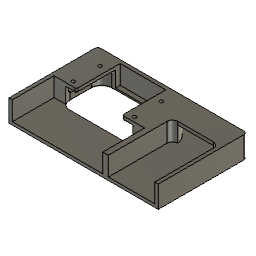
co2_o2_fascia (Autodesk Fusion 360 design; units mm, degrees)
part number: 2026-03-11-11-56-11-354
Autodesk Fusion 360 part; units mm, degrees
note: some values were not read from the file. Set by a fixed rule: which sketch regions a step uses.
sketch "Sketch1" plane through (0, 0, 0) normal (0, 0, 1) x (1, 0, 0)
  line L0 (0, 0) -> (95, 0)
  line L1 (95, 0) -> (95, 56.5)
  line L2 (95, 56.5) -> (0, 56.5)
  line L3 (0, 56.5) -> (0, 0)
  dimension "d1" = 95
  dimension "d2" = 56.5
  constraint horizontal L0
  constraint vertical L1
  constraint horizontal L2
  constraint vertical L3
  constraint coincident L0.start L3.end
  measures "d1" distance of L0.start L0.end
  measures "d2" distance of L0.start L2.end
extrude "Extrude1" add sketch "Sketch1" along normal blind 14
sketch "Sketch2" plane through (0, 0, 14) normal (0, 0, 1) x (-1, 0, 0)
  line L0 (0, -56.5) -> (0, 0)
  line L1 (0, 0) -> (-95, 0)
  line L2 (-95, 0) -> (-95, -56.5)
  line L3 (-95, -56.5) -> (0, -56.5)
  line L4 (-2.25, -26.5) -> (-92.75, -26.5)
  line L5 (-92.75, -26.5) -> (-92.75, 0.5)
  line L6 (-92.75, 0.5) -> (-2.25, 0.5)
  line L7 (-2.25, 0.5) -> (-2.25, -26.5)
  line L8 (-92.75, -26.5) -> (-60, -26.5)
  dimension "d5" = 90.5
  dimension "d6" = 27
  dimension "d7" = 30
  dimension "d8" = 2.25
  constraint horizontal L4
  constraint vertical L5
  constraint horizontal L6
  constraint vertical L7
  constraint horizontal L8
  measures "d5" distance of L4.start L4.end
  measures "d6" distance of L4.start L6.end
  measures "d7" distance of L3 L4
  measures "d8" distance of L0 L7
extrude "Extrude2" cut sketch "Sketch2" against normal blind 12 contours L1 L4 L5 L7 L8 | L1 L5 L6 L7
sketch "Sketch3" plane through (0, 0, 14) normal (0, 0, 1) x (-1, 0, 0)
  line L0 (-92.75, -26.5) -> (-92.75, 0)
  line L1 (-92.75, 0) -> (-95, 0)
  line L2 (-95, 0) -> (-95, -56.5)
  line L3 (-95, -56.5) -> (0, -56.5)
  line L4 (0, -56.5) -> (0, 0)
  line L5 (0, 0) -> (-2.25, 0)
  line L6 (-2.25, 0) -> (-2.25, -26.5)
  line L7 (-2.25, -26.5) -> (-92.75, -26.5)
  point P0 (-11.5, -46.5)
  point P1 (-50.5, -46.5)
  point P2 (-11.5, -29.5)
  point P3 (-50.5, -29.5)
  dimension "d11" = 10
  dimension "d12" = 11.5
  dimension "d15" = -39
  dimension "d16" = 17
  measures "d11" distance of L3 P0
  measures "d12" distance of L4 P0
hole "Hole1" at (50.5, 46.5, 14) at (50.5, 29.5, 14) at (11.5, 29.5, 14) at (11.5, 46.5, 14) direction (0, 0, -1) diameter 2.2 end through all
sketch "Sketch4" plane through (0, 0, 0) normal (0, 0, -1) x (1, 0, 0)
  circle A0 centre (11.5, -29.5) radius 1.1
  circle A1 centre (50.5, -46.5) radius 1.1
  circle A2 centre (50.5, -29.5) radius 1.1
  circle A3 centre (11.5, -46.5) radius 1.1
  line L0 (0, 0) -> (0, -56.5)
  line L1 (0, -56.5) -> (95, -56.5)
  line L2 (95, -56.5) -> (95, 0)
  line L3 (95, 0) -> (0, 0)
  line L4 (47.75, -51.275) -> (14.2, -51.275)
  line L5 (7.7, -44.775) -> (7.7, -31.225)
  line L6 (14.2, -24.725) -> (47.75, -24.725)
  line L7 (54.25, -31.225) -> (54.25, -44.775)
  arc A4 (47.75, -51.275) -> (54.25, -44.775) centre (47.75, -44.775) ccw
  arc A5 (7.7, -44.775) -> (14.2, -51.275) centre (14.2, -44.775) ccw
  arc A6 (14.2, -24.725) -> (7.7, -31.225) centre (14.2, -31.225) ccw
  arc A7 (54.25, -31.225) -> (47.75, -24.725) centre (47.75, -31.225) ccw
  point P0 (54.25, -51.275)
  point P1 (7.7, -51.275)
  point P2 (54.25, -24.725)
  dimension "d19" = 46.55
  dimension "d20" = 26.55
  dimension "d21" = 40.75
  dimension "d22" = 4.775
  dimension "d35" = 6.5
  constraint horizontal L4
  constraint vertical L5
  constraint horizontal L6
  constraint vertical L7
  constraint coincident P0 L7
  constraint coincident P0 L4
  constraint tangent L7 A4
  constraint tangent L4 A4
  constraint coincident P1 L4
  constraint coincident P1 L5
  constraint tangent L4 A5
  constraint tangent L5 A5
  constraint equal A4 A5
  constraint tangent L5 A6
  constraint tangent L6 A6
  constraint equal A4 A6
  constraint coincident P2 L6
  constraint coincident P2 L7
  constraint tangent L6 A7
  constraint tangent L7 A7
  constraint equal A4 A7
  measures "d19" distance of P0 P1
  measures "d20" distance of P0 P2
  measures "d21" distance of L2 L7
  measures "d22" distance of A1.centre L4
  measures "d35" radius of A4
extrude "Extrude3" cut sketch "Sketch4" against normal blind 11 contours L4 L5 L6 L7 A4 A5 A6 A7
sketch "Sketch5" plane through (0, 0, 0) normal (-1, 0, 0) x (0, -1, 0)
  line L0 (-56.5, 0) -> (0, 0)
  line L1 (0, 0) -> (0, 14)
  line L2 (0, 14) -> (-56.5, 14)
  line L3 (-56.5, 14) -> (-56.5, 0)
sketch "Sketch7" plane through (0, 0, 0) normal (-1, 0, 0) x (0, -1, 0)
  line L0 (-32, 13) -> (-44, 13)
  line L1 (-46, 11) -> (-46, 7)
  line L2 (-44, 5) -> (-32, 5)
  line L3 (-30, 7) -> (-30, 11)
  line L4 (-56.5, 14) -> (-56.5, 0)
  arc A0 (-32, 5) -> (-30, 7) centre (-32, 7) ccw
  arc A1 (-46, 7) -> (-44, 5) centre (-44, 7) ccw
  line L5 (-56.5, 0) -> (0, 0)
  arc A2 (-30, 11) -> (-32, 13) centre (-32, 11) ccw
  arc A3 (-44, 13) -> (-46, 11) centre (-44, 11) ccw
  point P0 (-30, 13)
  point P1 (-46, 13)
  point P2 (-30, 5)
  dimension "d30" = 16
  dimension "d31" = 8
  dimension "d32" = 10.5
  dimension "d42" = 2
  dimension "d140" = 5
  dimension "d141" = 2
  dimension "d142" = 2
  constraint horizontal L0
  constraint vertical L1
  constraint horizontal L2
  constraint vertical L3
  constraint coincident P2 L3
  constraint coincident P2 L2
  constraint tangent L3 A0
  constraint tangent L2 A0
  constraint tangent L2 A1
  constraint tangent L1 A1
  constraint equal A0 A1
  constraint coincident P0 L3
  constraint coincident P0 L0
  constraint tangent L3 A2
  constraint tangent L0 A2
  constraint coincident P1 L0
  constraint coincident P1 L1
  constraint tangent L0 A3
  constraint tangent L1 A3
  measures "d30" distance of P0 P1
  measures "d31" distance of P0 P2
  measures "d32" distance of L1 L4
  measures "d42" radius of A0
  measures "d140" distance of L2 L5
  measures "d141" radius of A2
  measures "d142" radius of A3
extrude "Extrude5" cut sketch "Sketch7" against normal blind 8.5
sketch "Sketch8" plane through (0, 0, 14) normal (0, 0, 1) x (-1, 0, 0)
  line L0 (0, 0) -> (-2.25, 0)
  line L1 (-2.25, 0) -> (-2.25, -26.5)
  line L2 (-2.25, -26.5) -> (-92.75, -26.5)
  line L3 (-92.75, -26.5) -> (-92.75, 0)
  line L4 (-92.75, 0) -> (-95, 0)
  line L5 (-95, 0) -> (-95, -56.5)
  line L6 (-95, -56.5) -> (0, -56.5)
  line L7 (0, -56.5) -> (0, 0)
  circle A0 centre (-11.5, -29.5) radius 1.1
  circle A1 centre (-50.5, -46.5) radius 1.1
  circle A2 centre (-50.5, -29.5) radius 1.1
  circle A3 centre (-11.5, -46.5) radius 1.1
  line L8 (-16.5, -54.25) -> (-45.5, -54.25)
  line L9 (-45.5, -54.25) -> (-45.5, -14.25)
  line L10 (-45.5, -14.25) -> (-16.5, -14.25)
  line L11 (-16.5, -14.25) -> (-16.5, -54.25)
  dimension "d36" = 29
  dimension "d37" = 40
  dimension "d38" = 2.25
  dimension "d39" = 49.5
  constraint horizontal L8
  constraint vertical L9
  constraint horizontal L10
  constraint vertical L11
  measures "d36" distance of L8.start L8.end
  measures "d37" distance of L8.start L10.end
  measures "d38" distance of L6 L8
  measures "d39" distance of L5 L9
extrude "Extrude6" cut sketch "Sketch8" against normal blind 2.5 contours L2 L8 L9 L11 | L2 L9 L10 L11
fillet "Fillet1" radius 2 1 edges at (95, 56.5, 7)
fillet "Fillet2" radius 2 1 edges at (0, 56.5, 7)
fillet "Fillet3" radius 1 8 edges at (7.7, 38, 0) (9.6038, 26.6288, 0) (30.975, 24.725, 0) (52.3462, 26.6288, 0) (54.25, 38, 0) (52.3462, 49.3712, 0) (30.975, 51.275, 0) (9.6038, 49.3712, 0)
fillet "Fillet4" radius 1 5 edges at (0, 30, 9) (0, 30.5858, 5.5858) (0, 38, 5) (0, 45.4142, 5.5858) (0, 46, 9)
extrude "Extrude13" cut 1 faces at (35.8333, 45, 11.5) along direction (0, 0, -1) blind 9.5
sketch "Sketch13" plane through (0, 0, 14) normal (0, 0, 1) x (-1, 0, 0)
  arc A0 (-2, -56.5) -> (0, -54.5) centre (-2, -54.5) ccw
  line L0 (0, -54.5) -> (0, -44)
  line L1 (0, 0) -> (-2.25, 0)
  line L2 (-2.25, 0) -> (-2.25, -26.5)
  line L3 (-2.25, -26.5) -> (-16.5, -26.5)
  line L4 (-16.5, -26.5) -> (-16.5, -54.25)
  line L5 (-16.5, -54.25) -> (-45.5, -54.25)
  line L6 (-45.5, -54.25) -> (-45.5, -26.5)
  line L7 (-45.5, -26.5) -> (-92.75, -26.5)
  line L8 (-92.75, -26.5) -> (-92.75, 0)
  line L9 (-92.75, 0) -> (-95, 0)
  line L10 (-95, 0) -> (-95, -54.5)
  arc A1 (-95, -54.5) -> (-93, -56.5) centre (-93, -54.5) ccw
  line L11 (-93, -56.5) -> (-2, -56.5)
  circle A2 centre (-11.5, -29.5) radius 1.1
  circle A3 centre (-50.5, -46.5) radius 1.1
  circle A4 centre (-50.5, -29.5) radius 1.1
  circle A5 centre (-11.5, -46.5) radius 1.1
  line L12 (-92.75, -26.5) -> (-63.25, -26.5)
  line L13 (-63.25, -26.5) -> (-63.25, -37.331)
  line L14 (-66.669, -40.75) -> (-89.331, -40.75)
  line L15 (-92.75, -37.331) -> (-92.75, -26.5)
  arc A6 (-66.669, -40.75) -> (-63.25, -37.331) centre (-66.669, -37.331) ccw
  arc A7 (-92.75, -37.331) -> (-89.331, -40.75) centre (-89.331, -37.331) ccw
  line L16 (0, -44) -> (0, -32)
  line L17 (0, -32) -> (0, 0)
  dimension "d107" = 29.5
  dimension "d108" = 15.75
  dimension "d118" = 3.419
  dimension "d119" = 3.419
  constraint horizontal L12
  constraint vertical L13
  constraint horizontal L14
  constraint vertical L15
  constraint coincident L7.end L8.start
  constraint tangent L13 A6
  constraint tangent L14 A6
  constraint tangent L14 A7
  constraint tangent L15 A7
  measures "d107" distance of L7.end L12.end
  measures "d108" distance of L11 L14
  measures "d118" radius of A6
  measures "d119" radius of A7
extrude "Extrude20" cut sketch "Sketch13" against normal blind 12 contours L7 L12 L13 L14 L15 A6 A7
sketch "Sketch16" plane through (0, 40.75, 0) normal (0, -1, 0) x (1, 0, 0)
  line L0 (89.331, 14) -> (66.669, 14)
  line L1 (66.669, 14) -> (66.669, 2)
  line L2 (66.669, 2) -> (89.331, 2)
  line L3 (89.331, 2) -> (89.331, 14)
  line L4 (89.331, 2) -> (66.669, 2)
  line L5 (66.669, 2) -> (66.669, 12)
  line L6 (66.669, 12) -> (89.331, 12)
  line L7 (89.331, 12) -> (89.331, 2)
  dimension "d120" = 10
  constraint horizontal L4
  constraint vertical L5
  constraint horizontal L6
  constraint vertical L7
  constraint coincident L1 L5.end
  constraint coincident L2.end L3.start
  measures "d120" distance of L2.end L6.end
extrude "Extrude23" cut sketch "Sketch16" against normal blind 13.5 contours L1 L2 L3 L4 L5 L6 L7
sketch "Sketch17" plane through (66.669, 0, 0) normal (1, 0, 0) x (0, 1, 0)
  line L0 (40.75, 12) -> (40.75, 2)
  line L1 (40.75, 2) -> (54.25, 2)
  line L2 (54.25, 2) -> (54.25, 12)
  line L3 (54.25, 12) -> (40.75, 12)
  line L4 (54.25, 2) -> (49.25, 2)
  line L5 (49.25, 2) -> (49.25, 12)
  line L6 (49.25, 12) -> (54.25, 12)
  line L7 (54.25, 12) -> (54.25, 2)
  dimension "d123" = 5
  dimension "d124" = 10
  constraint horizontal L4
  constraint vertical L5
  constraint horizontal L6
  constraint vertical L7
  constraint coincident L1.end L2.start
  measures "d123" distance of L1.end L4.end
  measures "d124" distance of L1.end L2.end
extrude "Extrude24" cut sketch "Sketch17" against normal blind 30 contours L1 L2 L3 L4 L5 L6 L7
fillet "Fillet15" radius 10 1 edges at (66.669, 49.25, 7)
sketch "Sketch18" plane through (0, 26.5, 0) normal (0, -1, 0) x (1, 0, 0)
  line L0 (63.25, 2) -> (63.25, 14)
  line L1 (63.25, 14) -> (45.5, 14)
  line L2 (45.5, 14) -> (45.5, 11)
  line L3 (45.5, 11) -> (52.2137, 11)
  line L4 (52.2137, 11) -> (52.2137, 2)
  line L5 (52.2137, 2) -> (63.25, 2)
  line L6 (59.75, 2) -> (63.25, 2)
  line L7 (63.25, 2) -> (63.25, 14)
  line L8 (63.25, 14) -> (59.75, 14)
  line L9 (59.75, 14) -> (59.75, 2)
  point P0 (0, 14)
  dimension "d129" = 59.75
  constraint horizontal L6
  constraint vertical L7
  constraint horizontal L8
  constraint vertical L9
  constraint coincident L0.end L1.start
  constraint coincident L5 L6.start
  measures "d129" distance of L9 P0
extrude "Extrude25" add sketch "Sketch18" along normal blind 26.5 contours L0 L1 L5 L6 L7 L8 L9
fillet "Fillet16" radius 1 1 edges at (45.5, 37.875, 11)
fillet "Fillet17" radius 1 1 edges at (16.5, 38.8875, 11)
fillet "Fillet18" radius 1 3 edges at (45.5, 26.5, 13) (45.7929, 26.5, 11.2929) (49.3568, 26.5, 11)
fillet "Fillet19" radius 1 3 edges at (12.6182, 26.5, 11) (16.2071, 26.5, 11.2929) (16.5, 26.5, 13)
sketch "Sketch19" plane through (0, 0, 0) normal (0, 0, -1) x (1, 0, 0)
  arc A0 (0, -54.5) -> (2, -56.5) centre (2, -54.5) ccw
  line L0 (2, -56.5) -> (93, -56.5)
  arc A1 (93, -56.5) -> (95, -54.5) centre (93, -54.5) ccw
  line L1 (95, -54.5) -> (95, 0)
  line L2 (95, 0) -> (0, 0)
  line L3 (0, 0) -> (0, -54.5)
  line L4 (6.7, -44.775) -> (6.7, -31.225)
  arc A2 (14.2, -23.725) -> (6.7, -31.225) centre (14.2, -31.225) ccw
  line L5 (14.2, -23.725) -> (47.75, -23.725)
  arc A3 (55.25, -31.225) -> (47.75, -23.725) centre (47.75, -31.225) ccw
  line L6 (55.25, -31.225) -> (55.25, -44.775)
  arc A4 (47.75, -52.275) -> (55.25, -44.775) centre (47.75, -44.775) ccw
  line L7 (47.75, -52.275) -> (14.2, -52.275)
  arc A5 (6.7, -44.775) -> (14.2, -52.275) centre (14.2, -44.775) ccw
  line L8 (90.1582, -3.3158) -> (49.1582, -3.3158) construction
  line L9 (49.1582, -3.3158) -> (49.1582, -16.3158) construction
  line L10 (49.1582, -16.3158) -> (90.1582, -16.3158) construction
  line L11 (90.1582, -16.3158) -> (90.1582, -3.3158) construction
  dimension "d143" = 10
  text T0 "Bamako" font "Arial" height 10 bold align left top in box 41 x 13 at (90.1582, -3.3158) x (-1, 0) y (0, -1) spacing 1
extrude "Extrude26" add sketch "Sketch19" along normal blind 0.0001 text T0
equation "d144 = 'Bamako'"
